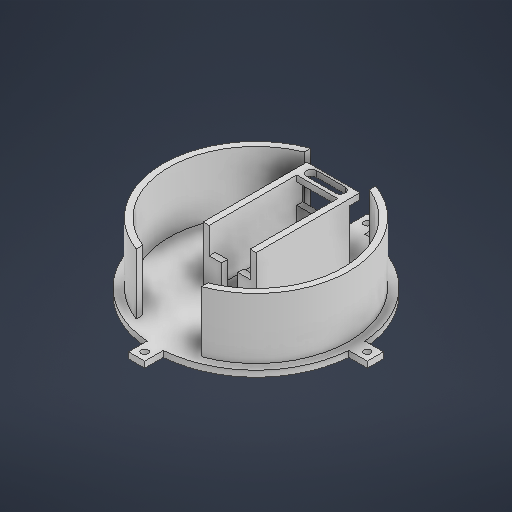
# Autodesk Inventor part: spinny base
Saved by Autodesk Inventor 2026.1 (Build 301233000, 233)
## iProperties
Created: 2025-10-15
Part Number: spinny base
Material: Generic
Document SubType Name: Modeling
Designer: Ethan
Density: 1 g/cm^3
Appearance: Default
Author: Ethan
Autodesk Inventor part; units mm, degrees
ref_plane "YZ Plane" through (0, 0, 0) normal (1, 0, 0) x (0, 1, 0)
ref_plane "XZ Plane" through (0, 0, 0) normal (0, 1, 0) x (-1, 0, 0)
ref_plane "XY Plane" through (0, 0, 0) normal (0, 0, 1) x (1, 0, 0)
sketch "Sketch1" plane through (0, 0, 0) normal (0, 1, 0) x (-1, 0, 0)
  circle A0 centre (0, 0) radius 70.5
  circle A1 centre (0, 0) radius 75.5
  dimension "d0" = 141
  dimension "d4" = 5
  constraints: 2 centre point, 1 coincident
  measures "d0" diameter of A0
  measures "d4" radial gap between concentric circles of A0 A1
extrude "Extrusion1" add sketch "Sketch1" along normal blind 50
sketch "Sketch2" plane through (0, 0, 0) normal (0, -1, 0) x (1, 0, 0)
  line L0 (-10.125, 10) -> (10.125, 10)
  line L1 (10.125, 10) -> (10.125, -30.25)
  line L2 (10.125, -30.25) -> (-10.125, -30.25)
  line L3 (-10.125, -30.25) -> (-10.125, 10)
  point P0 (0, 0)
  point P1 (0, 10)
  dimension "d5" = 20.25
  dimension "d6" = 40.25
  dimension "d7" = 10
  dimension "d8" = 10.125
  dimension "d9" = 10.125
  constraints: 8 end point, 2 parallel, 1 horizontal, 1 midpoint, 1 perpendicular
  measures "d5" distance of L1.end L2.end
  measures "d6" distance of L2.end L0.start
  measures "d7" distance of point (0, 0) point (0, 10)
  measures "d8" distance from line of point (0, 0) L1
  measures "d9" distance from line of point (0, 0) L3
extrude "Extrusion2" add sketch "Sketch2" against normal blind 3
sketch "Sketch3" plane through (0, 0, 0) normal (0, -1, 0) x (1, 0, 0)
  line L0 (13.125, 13) -> (10.125, 13)
  line L1 (10.125, 13) -> (10.125, -33.25)
  line L2 (10.125, -33.25) -> (13.125, -33.25)
  line L3 (13.125, -33.25) -> (13.125, 13)
  line L4 (10.125, -33.25) -> (-13.125, -33.25)
  line L5 (-13.125, -33.25) -> (-13.125, -30.25)
  line L6 (-13.125, -30.25) -> (10.125, -30.25)
  line L7 (10.125, -30.25) -> (10.125, -33.25)
  line L8 (-13.125, -30.25) -> (-10.125, -30.25)
  line L9 (-10.125, -30.25) -> (-10.125, 13)
  line L10 (-10.125, 13) -> (-13.125, 13)
  line L11 (-13.125, 13) -> (-13.125, -30.25)
  line L12 (-10.125, -30.25) -> (10.125, -30.25) projected
  line L13 (10.125, -30.25) -> (10.125, 10) projected
  line L14 (-10.125, 10) -> (-10.125, -30.25) projected
  line L15 (10.125, 10) -> (-10.125, 10) projected
  line L16 (10.125, 13) -> (4, 13)
  line L17 (4, 13) -> (4, 10)
  line L18 (4, 10) -> (10.125, 10)
  line L19 (10.125, 10) -> (10.125, 13)
  line L20 (-10.125, 13) -> (-4, 13)
  line L21 (-4, 13) -> (-4, 10)
  line L22 (-4, 10) -> (-10.125, 10)
  line L23 (-10.125, 10) -> (-10.125, 13)
  point P0 (0, 0)
  point P1 (-11.625, 13)
  point P2 (10.125, 11.5)
  dimension "d12" = 3
  dimension "d13" = 3
  dimension "d14" = 3
  dimension "d15" = 0
  dimension "d16" = 0
  dimension "d17" = 0
  dimension "d18" = 3
  dimension "d19" = 3
  dimension "d20" = 6.125
  dimension "d21" = 6.125
  constraints: 40 end point, 10 parallel, 5 horizontal, 5 perpendicular, 2 midpoint, 2 point on line
  measures "d12" distance between parallel lines of L3 L1
  measures "d13" distance between parallel lines of L4 L6
  measures "d14" distance between parallel lines of L9 L11
  measures "d15" distance between parallel lines of L12 L6
  measures "d16" distance between parallel lines of L1 L13
  measures "d17" distance between parallel lines of L14 L9
  measures "d18" distance from line of L15 point (-11.625, 13)
  measures "d19" distance between parallel lines of L15 L0
  measures "d20" distance of L9.end L20.end
  measures "d21" distance from line of point (10.125, 11.5) L17
extrude "Extrusion3" add sketch "Sketch3" against normal blind 18 contours L3 L2 L1 L0 | L1 L15 L17 L16 | L4 L5 L6 L1 | L6 L11 L10 L9 | L15 L9 L20 L21
sketch "Sketch4" plane through (0, 18, 0) normal (0, 1, 0) x (1, 0, 0)
  line L0 (-4, -13) -> (-13.125, -13) projected
  line L1 (-13.125, 33.25) -> (13.125, 33.25) projected
  line L2 (-13.125, -13) -> (-10.125, -13)
  line L3 (-10.125, -13) -> (-10.125, 33.25)
  line L4 (-10.125, 33.25) -> (-13.125, 33.25)
  line L5 (-13.125, 33.25) -> (-13.125, -13)
  line L6 (13.125, -13) -> (13.125, 33.25) projected
  line L7 (13.125, 33.25) -> (10.125, 33.25)
  line L8 (10.125, 33.25) -> (10.125, -13)
  line L9 (10.125, -13) -> (13.125, -13)
  line L10 (13.125, -13) -> (13.125, 33.25)
  line L11 (-10.125, -10) -> (-10.125, 30.25) projected
  point P0 (0, 0)
  dimension "d24" = 0
  constraints: 16 end point, 4 parallel, 2 horizontal, 2 perpendicular, 2 point on line
  measures "d24" distance between parallel lines of L11 L3
extrude "Extrusion4" add sketch "Sketch4" along normal blind 13
sketch "Sketch5" plane through (13.125, 0, -33.25) normal (0, 0, -1) x (-1, 0, 0)
  line L0 (23.25, 31) -> (26.25, 31) projected
  line L1 (0, 0) -> (0, 31) projected
  line L2 (26.25, 31) -> (0, 31)
  line L3 (0, 31) -> (0, 28)
  line L4 (0, 28) -> (26.25, 28)
  line L5 (26.25, 28) -> (26.25, 31)
  point P0 (13.125, 0)
  dimension "d27" = 3
  constraints: 8 end point, 2 parallel, 1 horizontal, 1 perpendicular, 1 point on line
  measures "d27" distance between parallel lines of L2 L4
extrude "Extrusion5" add sketch "Sketch5" along normal blind 5
sketch "Sketch6" plane through (0, 31, 0) normal (0, 1, 0) x (1, 0, 0)
  line L0 (10.125, 33.25) -> (-10.125, 33.25) projected
  line L1 (-10.125, 33.25) -> (10.125, 33.25)
  line L2 (10.125, 33.25) -> (10.125, 30.25)
  line L3 (10.125, 30.25) -> (-10.125, 30.25)
  line L4 (-10.125, 30.25) -> (-10.125, 33.25)
  point P0 (0, 0)
  constraints: 8 end point, 2 parallel, 1 horizontal, 1 perpendicular
extrude "Extrusion6" add sketch "Sketch6" against normal blind 3
sketch "Sketch7" plane through (0, 31, 0) normal (0, 1, 0) x (1, 0, 0)
  circle A0 centre (-7.125, 34.55) radius 2.5
  circle A1 centre (7.125, 34.55) radius 2.5
  line L0 (-10.125, 30.25) -> (10.125, 30.25) projected
  line L1 (-13.125, -13) -> (-13.125, 38.25) projected
  line L2 (13.125, -13) -> (13.125, 38.25) projected
  line L3 (-7.125, 32.05) -> (7.125, 32.05)
  line L4 (7.125, 37.05) -> (-7.125, 37.05)
  point P0 (0, 0)
  dimension "d32" = 4.3
  dimension "d33" = 0
  dimension "d34" = 5
  dimension "d35" = 5
  dimension "d36" = 6
  dimension "d37" = 6
  constraints: 4 end point, 4 point on circle, 2 centre point, 2 tangent, 1 parallel
  measures "d32" distance from line of L0 A0.centre
  measures "d33" vertical distance of A1.centre A0.centre
  measures "d34" diameter of A0
  measures "d35" diameter of A1
  measures "d36" distance from line of L1 A0.centre
  measures "d37" distance from line of L2 A1.centre
extrude "Extrusion7" cut sketch "Sketch7" against normal blind 3
sketch "Sketch8" plane through (0, 0, 0) normal (0, -1, 0) x (1, 0, 0)
  line L0 (72.6444, -3) -> (-73.2822, -3)
  line L1 (-73.2822, -3) -> (-73.2822, 3)
  line L2 (-73.2822, 3) -> (72.6444, 3)
  line L3 (72.6444, 3) -> (72.6444, -3)
  line L4 (3, -73.2385) -> (-3, -73.2385)
  line L5 (-3, -73.2385) -> (-3, 72.5895)
  line L6 (-3, 72.5895) -> (3, 72.5895)
  line L7 (3, 72.5895) -> (3, -73.2385)
  point P0 (0, 0)
  point P1 (-0.3189, -3)
  point P2 (3, -3)
  point P3 (3, 3)
  point P4 (-3, 3)
  point P5 (-3, -3)
  dimension "d40" = 3
  dimension "d41" = 3
  dimension "d42" = 3
  dimension "d43" = 3
  constraints: 16 end point, 4 parallel, 2 horizontal, 2 perpendicular, 1 midpoint
  measures "d40" vertical distance of point (-0.319, -3) point (0, 0)
  measures "d41" distance from line of point (0, 0) L2
  measures "d42" distance from line of point (0, 0) L7
  measures "d43" distance from line of point (0, 0) L5
extrude "Extrusion8" add sketch "Sketch8" against normal blind 3
sketch "Sketch9" plane through (0, 50, 0) normal (0, 1, 0) x (1, 0, 0)
  arc A0 (-3, 70.4361) -> (-70.4361, 3) centre (0, 0) ccw projected
  line L0 (-15, 68.8858) -> (15, 68.8858)
  circle A1 centre (0, 0) radius 70.5 projected
  line L1 (-68.8858, -15) -> (-68.8858, 15)
  line L2 (15, -68.8858) -> (-15, -68.8858)
  line L3 (68.8858, 15) -> (68.8858, -15)
  dimension "d46" = 30
  dimension "d49" = 360
  constraints: 8 end point, 2 point on circle, 1 horizontal, 13 other
  measures "d46" distance of L0.start L0.end
extrude "Extrusion9" add sketch "Sketch9" against normal blind 50 contours A1 L0 A0 | L1 A1 A0 | A1 L3 | L2 A1
sketch "Sketch10" plane through (-68.8858, 50, 15) normal (1, 0, 0) x (0, 0, -1)
  circle A0 centre (15, -12) radius 5
  line L0 (45.25, -47) -> (5, -47) projected
  line L1 (0, -50) -> (0, 0) projected
  point P0 (15, -50)
  dimension "d53" = 10
  dimension "d54" = 35
  dimension "d55" = 15
  constraints: 1 centre point
  measures "d53" diameter of A0
  measures "d54" distance from line of A0.centre L0
  measures "d55" distance from line of L1 A0.centre
sketch "Sketch11" plane through (0, 3, 0) normal (0, 1, 0) x (1, 0, 0)
  point P0 (0, 0)
extrude "Extrusion10" add sketch "Sketch10" along normal blind 2
sketch "Sketch12" plane through (-66.8858, 38, 0) normal (1, 0, 0) x (0, 0, -1)
  circle A0 centre (0, 0) radius 3.97
  point P0 (0, -38)
  dimension "d58" = 7.94
  constraints: 1 centre point
  measures "d58" diameter of A0
extrude "Extrusion11" add sketch "Sketch12" along normal blind 11
sketch "Sketch13" plane through (-15, 50, -68.8858) normal (0, 0, 1) x (1, 0, 0)
  circle A0 centre (15, -12) radius 5
  line L0 (25.125, -47) -> (4.875, -47) projected
  point P0 (15, -50)
  dimension "d61" = 10
  dimension "d62" = 35
  constraints: 1 centre point
  measures "d61" diameter of A0
  measures "d62" distance from line of L0 A0.centre
extrude "Extrusion12" add sketch "Sketch13" along normal blind 2
sketch "Sketch14" plane through (0, 38, -66.8858) normal (0, 0, 1) x (1, 0, 0)
  circle A0 centre (0, 0) radius 5 projected
  circle A1 centre (0, 0) radius 3.97
  point P0 (0, -38)
  dimension "d65" = 7.94
  constraints: 1 centre point, 1 coincident
  measures "d65" diameter of A1
extrude "Extrusion13" add sketch "Sketch14" along normal blind 11 contours A1
sketch "Sketch15" plane through (68.8858, 50, -15) normal (-1, 0, 0) x (0, 0, 1)
  circle A0 centre (15, -12) radius 5
  line L0 (25, -47) -> (-15.25, -47) projected
  point P0 (15, -50)
  dimension "d68" = 10
  dimension "d69" = 35
  constraints: 1 centre point
  measures "d68" diameter of A0
  measures "d69" distance from line of A0.centre L0
extrude "Extrusion14" add sketch "Sketch15" along normal blind 2
sketch "Sketch16" plane through (66.8858, 38, 0) normal (-1, 0, 0) x (0, 0, 1)
  circle A0 centre (0, 0) radius 3.97
  point P0 (0, -38)
  dimension "d72" = 7.94
  constraints: 1 centre point
  measures "d72" diameter of A0
extrude "Extrusion15" add sketch "Sketch16" along normal blind 11
sketch "Sketch17" plane through (15, 50, 68.8858) normal (0, 0, -1) x (-1, 0, 0)
  circle A0 centre (15, -12) radius 5
  line L0 (12, -47) -> (11, -47) projected
  point P0 (15, -50)
  point P1 (11.5, -47)
  dimension "d75" = 10
  dimension "d76" = 35
  constraints: 1 centre point, 1 midpoint
  measures "d75" diameter of A0
  measures "d76" vertical distance of point (11.5, -47) A0.centre
extrude "Extrusion16" add sketch "Sketch17" along normal blind 2
sketch "Sketch18" plane through (0, 38, 66.8858) normal (0, 0, -1) x (-1, 0, 0)
  circle A0 centre (0, 0) radius 5 projected
  circle A1 centre (0, 0) radius 3.97
  point P0 (0, -38)
  dimension "d79" = 7.94
  constraints: 1 centre point, 1 coincident
  measures "d79" diameter of A1
extrude "Extrusion17" add sketch "Sketch18" along normal blind 11 contours A1
sketch "Sketch19" plane through (0, 50, 0) normal (0, 1, 0) x (1, 0, 0)
  circle A0 centre (0, 0) radius 70.5
  constraints: 1 centre point, 1 coincident
extrude "Extrusion18" cut sketch "Sketch19" against normal blind 8
sketch "Sketch20" plane through (0, 50, 0) normal (0, 1, 0) x (1, 0, 0)
  circle A0 centre (0, 0) radius 75.5
  circle A1 centre (0, 0) radius 70.5
  constraints: 2 centre point, 2 coincident
extrude "Extrusion19" add sketch "Sketch20" along normal blind 10
sketch "Sketch21" plane through (15, 0, 68.8858) normal (0, 0, -1) x (-1, 0, 0)
  line L0 (18, 0) -> (18, 3) projected
  line L1 (18, 3) -> (13, 3)
  line L2 (13, 3) -> (13, 16.2196)
  line L3 (13, 16.2196) -> (18, 16.2196)
  line L4 (18, 16.2196) -> (18, 3)
  point P0 (15, 0)
  dimension "d87" = 5
  dimension "d88" = 13.2196
  constraints: 8 end point, 2 parallel, 1 horizontal, 1 perpendicular
  measures "d87" distance between parallel lines of L4 L2
  measures "d88" distance of L3.end L0.end
extrude "Extrusion20" cut sketch "Sketch21" against normal blind 10
sketch "Sketch22" plane through (0, 60, 0) normal (0, 1, 0) x (1, 0, 0)
  circle A0 centre (0, 0) radius 75.5 projected
  line L0 (-59.9939, -45.8364) -> (-80.9066, -64.8839)
  line L1 (-80.9066, -64.8839) -> (-67.4393, -79.67)
  line L2 (-67.4393, -79.67) -> (-45.8364, -59.9939)
  line L3 (-45.8364, -59.9939) -> (-59.9939, -45.8364)
  line L4 (-66.8858, -5) -> (-66.8858, 5) projected
  line L5 (64.8839, -80.9066) -> (79.67, -67.4393)
  line L6 (79.67, -67.4393) -> (59.9939, -45.8364)
  line L7 (45.8364, -59.9939) -> (64.8839, -80.9066)
  line L8 (59.9939, -45.8364) -> (45.8364, -59.9939)
  line L9 (80.9066, 64.8839) -> (67.4393, 79.67)
  line L10 (67.4393, 79.67) -> (45.8364, 59.9939)
  line L11 (59.9939, 45.8364) -> (80.9066, 64.8839)
  line L12 (45.8364, 59.9939) -> (59.9939, 45.8364)
  line L13 (-64.8839, 80.9066) -> (-79.67, 67.4393)
  line L14 (-79.67, 67.4393) -> (-59.9939, 45.8364)
  line L15 (-45.8364, 59.9939) -> (-64.8839, 80.9066)
  line L16 (-59.9939, 45.8364) -> (-45.8364, 59.9939)
  point P0 (-52.9152, -52.9152)
  point P1 (52.9152, -52.9152)
  point P2 (52.9152, 52.9152)
  point P3 (-52.9152, 52.9152)
  dimension "d91" = 45
  dimension "d92" = 20
  dimension "d93" = 52.9152
  dimension "d96" = 360
  constraints: 32 end point, 2 perpendicular, 2 point on circle, 1 midpoint, 37 other
  measures "d91" angle of L4 L3
  measures "d92" distance between parallel lines of L2 L0
  measures "d93" horizontal distance of point (0, 0) point (-52.915, -52.915)
extrude "Extrusion21" add sketch "Sketch22" against normal blind 60 contours A0 L10 L9 L11 | L6 L5 L7 A0 | A0 L8 | A0 L14 L13 L15 | L2 L1 L0 A0
sketch "Sketch23" plane through (0, 60, 0) normal (0, 1, 0) x (1, 0, 0)
  arc A0 (-45.8364, -59.9939) -> (45.8364, -59.9939) centre (0, 0) ccw projected
  circle A1 centre (0, 0) radius 75.5
  line L0 (48.1887, -58.1214) -> (67.1018, -78.8865)
  line L1 (64.8839, -80.9066) -> (79.67, -67.4393) projected
  line L2 (78.1665, -70.2437) -> (58.101, -48.2133)
  line L3 (79.67, -67.4393) -> (59.9939, -45.8364) projected
  line L4 (45.8364, -59.9939) -> (64.8839, -80.9066) projected
  line L5 (67.1018, -78.8865) -> (61.0649, -93.7796)
  line L6 (61.0649, -93.7796) -> (42.6475, -67.861)
  line L7 (42.6475, -67.861) -> (45.8364, -59.9939)
  line L8 (67.1018, -78.8865) -> (77.4521, -69.4594)
  line L9 (58.1214, 48.1887) -> (78.8865, 67.1018)
  line L10 (70.2437, 78.1665) -> (48.2133, 58.101)
  line L11 (78.8865, 67.1018) -> (69.4594, 77.4521)
  circle A2 centre (0, 0) radius 75.5
  line L12 (-48.1887, 58.1214) -> (-67.1018, 78.8865)
  line L13 (-78.1665, 70.2437) -> (-58.101, 48.2133)
  line L14 (-67.1018, 78.8865) -> (-77.4521, 69.4594)
  circle A3 centre (0, 0) radius 75.5
  line L15 (-58.1214, -48.1887) -> (-78.8865, -67.1018)
  line L16 (-70.2437, -78.1665) -> (-48.2133, -58.101)
  line L17 (-78.8865, -67.1018) -> (-69.4594, -77.4521)
  circle A4 centre (0, 0) radius 75.5
  point P0 (45.8364, 59.9939)
  point P1 (-59.9939, 45.8364)
  point P2 (-45.8364, -59.9939)
  dimension "d100" = 3
  dimension "d101" = 3
  dimension "d102" = 151
  dimension "d105" = 360
  constraints: 30 end point, 8 point on circle, 7 point on line, 4 centre point, 3 parallel, 1 coincident, 49 other
  measures "d100" distance between parallel lines of L4 L0
  measures "d101" distance between parallel lines of L3 L2
  measures "d102" diameter of A1
extrude "Extrusion22" cut sketch "Sketch23" against normal blind 57 contours L16 L17 L15 A1 | A1 L2 L1 L0 | L13 L14 L12 A1 | L10 L11 L9 A1
sketch "Sketch24" plane through (59.9939, 0, -45.8364) normal (0.673368, 0, 0.7393075) x (0.7393075, 0, -0.673368)
  line L0 (0, 60) -> (-61.7295, 60) projected
  line L1 (28.2869, 0) -> (0, 0) projected
  line L2 (0, 60) -> (28.2869, 0)
  arc A0 (28.2869, 0) -> (0, 60) centre (28.2869, 36.6679) ccw
  point P0 (-75.2187, 0)
  constraints: 2 end point, 2 point on circle, 1 centre point, 1 tangent
extrude "Extrusion23" cut sketch "Sketch24" against normal blind 57
sketch "Sketch25" plane through (-45.8364, 0, -59.9939) normal (0.7393075, 0, -0.673368) x (-0.673368, 0, -0.7393075)
  line L0 (0.2813, 60) -> (-0.4509, 60) projected
  line L1 (-0.9335, 0) -> (28.2869, 0) projected
  line L2 (-0.4509, 60) -> (28.2869, 0)
  arc A0 (28.2869, 0) -> (-0.4509, 60) centre (28.2869, 36.8822) ccw
  point P0 (-75.2187, 0)
  point P1 (0.1996, 60)
  constraints: 2 end point, 2 point on circle, 1 centre point, 1 tangent
extrude "Extrusion24" cut sketch "Sketch25" against normal blind 57
sketch "Sketch26" plane through (-59.9939, 0, 45.8364) normal (-0.673368, 0, -0.7393075) x (-0.7393075, 0, 0.673368)
  line L0 (0, 0) -> (-61.7295, 0) projected
  line L1 (-0.9335, 0) -> (28.2869, 0) projected
  line L2 (0, 0) -> (28.2869, 0)
  arc A0 (28.2869, 0) -> (0, 67.3564) centre (28.2869, 39.6179) ccw
  line L3 (0, 67.3564) -> (0, 59.5281)
  line L4 (28.2869, 60) -> (28.2869, 0) projected
  line L5 (0, 59.5281) -> (28.2869, 0)
  point P0 (-75.2187, 0)
  constraints: 6 end point, 2 point on circle, 1 centre point, 1 collinear, 1 perpendicular, 1 tangent
extrude "Extrusion25" cut sketch "Sketch26" against normal blind 57
sketch "Sketch27" plane through (45.8364, 0, 59.9939) normal (-0.7393075, 0, 0.673368) x (0.673368, 0, 0.7393075)
  line L0 (0, 0) -> (0, 60) projected
  line L1 (28.2869, 0) -> (0, 0) projected
  line L2 (0, 60) -> (28.2869, 0)
  arc A0 (28.2869, 0) -> (0, 60) centre (28.2869, 36.6679) ccw
  point P0 (-75.2187, 0)
  constraints: 2 end point, 2 point on circle, 1 centre point, 1 tangent
extrude "Extrusion26" cut sketch "Sketch27" against normal blind 57 contours A0 L2
sketch "Sketch28" plane through (0, 3, 0) normal (0, 1, 0) x (1, 0, 0)
  circle A0 centre (67.6211, -69.0611) radius 2.5
  line L0 (66.1494, -77.8409) -> (76.4997, -68.4138) projected
  line L1 (76.4997, -68.4138) -> (58.4046, -48.5467) projected
  line L2 (48.1887, -58.1214) -> (66.1494, -77.8409) projected
  circle A1 centre (69.0611, 67.6211) radius 2.5
  circle A2 centre (-67.6211, 69.0611) radius 2.5
  circle A3 centre (-69.0611, -67.6211) radius 2.5
  point P0 (0, 0)
  dimension "d117" = 5
  dimension "d118" = 5.5
  dimension "d119" = 7
  dimension "d120" = 7
  dimension "d123" = 360
  constraints: 4 centre point, 9 other
  measures "d117" diameter of A0
  measures "d118" distance from line of L0 A0.centre
  measures "d119" distance from line of L1 A0.centre
  measures "d120" distance from line of L2 A0.centre
extrude "Extrusion27" cut sketch "Sketch28" against normal blind 57
sketch "Sketch29" plane through (0, 60, 0) normal (0, 1, 0) x (1, 0, 0)
  line L0 (-13.125, -13) -> (-13.125, -3) projected
  line L1 (13.125, -13) -> (13.125, 38.25) projected
  line L2 (-13.125, -13) -> (13.125, -13)
  line L3 (13.125, -13) -> (13.125, 38.25)
  line L4 (13.125, 38.25) -> (-13.125, 38.25)
  line L5 (-13.125, 38.25) -> (-13.125, -13)
  line L6 (-173.1074, 171.3287) -> (429.6424, 171.3287)
  line L7 (429.6424, 171.3287) -> (429.6424, -291.0697)
  line L8 (429.6424, -291.0697) -> (-173.1074, -291.0697)
  line L9 (-173.1074, -291.0697) -> (-173.1074, 171.3287)
  point P0 (0, 0)
  point P1 (-13.125, -3)
  constraints: 16 end point, 4 parallel, 2 horizontal, 2 perpendicular
extrude "Extrusion28" cut sketch "Sketch29" against normal blind 1111
sketch "Sketch30" plane through (0, 3, 0) normal (0, 1, 0) x (1, 0, 0)
  line L0 (3, 33.25) -> (-3, 33.25) projected
  line L1 (-3, 38.25) -> (-3, 33.25) projected
  line L2 (3, 33.25) -> (-3, 33.25)
  line L3 (-3, 33.25) -> (-3, 38.25)
  line L4 (-3, 38.25) -> (3, 38.25)
  line L5 (3, 38.25) -> (3, 33.25)
  point P0 (0, 0)
  constraints: 8 end point, 2 parallel, 1 horizontal, 1 perpendicular
extrude "Extrusion29" cut sketch "Sketch30" against normal blind 1111
sketch "Sketch31" plane through (0, 0, 0) normal (0, -1, 0) x (1, 0, 0)
  circle A0 centre (0, 0) radius 50
  dimension "d131" = 100
  constraints: 1 centre point, 1 coincident
  measures "d131" diameter of A0
extrude "Extrusion30" add sketch "Sketch31" against normal blind 3
sketch "Sketch32" plane through (0, 3, 0) normal (0, 1, 0) x (1, 0, 0)
  circle A0 centre (0, 0) radius 46
  circle A1 centre (0, 0) radius 43
  dimension "d134" = 92
  dimension "d135" = 3
  constraints: 2 centre point, 1 coincident
  measures "d134" diameter of A0
  measures "d135" radial gap between concentric circles of A0 A1
extrude "Extrusion31" add sketch "Sketch32" along normal blind 30
sketch "Sketch33" plane through (0, 33, 0) normal (0, 1, 0) x (1, 0, 0)
  line L0 (-16.125, 38.25) -> (16.125, 38.25)
  line L1 (16.125, 38.25) -> (16.125, 55.4979)
  line L2 (16.125, 55.4979) -> (-16.125, 55.4979)
  line L3 (-16.125, 55.4979) -> (-16.125, 38.25)
  line L4 (-13.125, -13) -> (-13.125, 38.25) projected
  line L5 (13.125, -13) -> (13.125, 38.25) projected
  line L6 (-16.125, -53.5102) -> (16.125, -53.5102)
  line L7 (16.125, -53.5102) -> (16.125, -24.6869)
  line L8 (16.125, -24.6869) -> (-16.125, -24.6869)
  line L9 (-16.125, -24.6869) -> (-16.125, -53.5102)
  point P0 (0, 0)
  dimension "d138" = 3
  dimension "d139" = 3
  constraints: 16 end point, 4 parallel, 2 horizontal, 2 perpendicular
  measures "d138" distance between parallel lines of L4 L3
  measures "d139" distance between parallel lines of L5 L1
extrude "Extrusion32" cut sketch "Sketch33" against normal blind 30
sketch "Sketch34" plane through (0, 0, 0) normal (0, -1, 0) x (1, 0, 0)
  circle A0 centre (0, 0) radius 50
  line L0 (49.9711, 1.7) -> (55, 1.7)
  line L1 (55, 1.7) -> (55, -1.7)
  line L2 (55, -1.7) -> (49.9711, -1.7)
  circle A1 centre (55, 0) radius 1.7
  line L3 (49.8397, 4) -> (59, 4)
  line L4 (59, 4) -> (59, -4)
  line L5 (59, -4) -> (49.8397, -4)
  circle A2 centre (0, 0) radius 50
  line L6 (-1.7, 49.9711) -> (-1.7, 55)
  line L7 (-1.7, 55) -> (1.7, 55)
  line L8 (1.7, 55) -> (1.7, 49.9711)
  circle A3 centre (0, 55) radius 1.7
  line L9 (-4, 49.8397) -> (-4, 59)
  line L10 (-4, 59) -> (4, 59)
  line L11 (4, 59) -> (4, 49.8397)
  circle A4 centre (0, 0) radius 50
  line L12 (-49.9711, -1.7) -> (-55, -1.7)
  line L13 (-55, -1.7) -> (-55, 1.7)
  line L14 (-55, 1.7) -> (-49.9711, 1.7)
  circle A5 centre (-55, 0) radius 1.7
  line L15 (-49.8397, -4) -> (-59, -4)
  line L16 (-59, -4) -> (-59, 4)
  line L17 (-59, 4) -> (-49.8397, 4)
  circle A6 centre (0, 0) radius 50
  line L18 (1.7, -49.9711) -> (1.7, -55)
  line L19 (1.7, -55) -> (-1.7, -55)
  line L20 (-1.7, -55) -> (-1.7, -49.9711)
  circle A7 centre (0, -55) radius 1.7
  line L21 (4, -49.8397) -> (4, -59)
  line L22 (4, -59) -> (-4, -59)
  line L23 (-4, -59) -> (-4, -49.8397)
  dimension "d142" = 3.4
  dimension "d143" = 100
  dimension "d144" = 55
  dimension "d145" = 0
  dimension "d146" = 4
  dimension "d147" = 4
  dimension "d148" = 4
  dimension "d151" = 360
  constraints: 48 end point, 16 point on circle, 4 centre point, 4 perpendicular, 2 horizontal, 2 horizontal alignment, 2 vertical alignment, 1 coincident, 1 midpoint, 81 other
  measures "d143" diameter of A0
  measures "d144" distance of point (0, 0) point (55, 0)
  measures "d145" vertical distance of point (0, 0) point (55, 0)
  measures "d146" distance from line of point (55, 0) L5
  measures "d147" distance from line of point (55, 0) L3
  measures "d148" distance from line of point (55, 0) L4
extrude "Extrusion33" add sketch "Sketch34" against normal blind 3 contours A0 L0 A1 L2 | A0 L3 L4 L5 L2 A1 L0 | A0 L8 A3 L6 L9 L10 L11 | L21 L22 L23 A0 L20 A7 L18 | A0 L6 A3 L8 | L18 A7 L20 A0 | A0 L14 A5 L12 L15 L16 L17 | A0 L12 A5 L14
body "Solid1"
